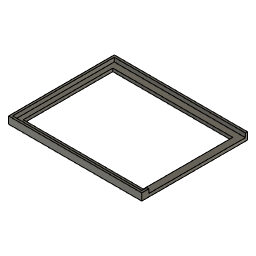
FrontPanel (Autodesk Fusion 360 design; units mm, degrees)
Autodesk Fusion 360 part; units mm, degrees
sketch "Sketch2" plane through (0, 0, 0) normal (0, 0, 1) x (1, 0, 0)
  line L0 (-55.8718, 52.373) -> (71.1282, 52.373)
  line L1 (71.1282, 52.373) -> (71.1282, -47.627)
  line L2 (71.1282, -47.627) -> (-55.8718, -47.627)
  line L3 (-55.8718, -47.627) -> (-55.8718, 52.373)
  line L4 (-51.3718, 46.373) -> (66.6282, 46.373)
  line L5 (66.6282, 46.373) -> (66.6282, -41.627)
  line L6 (66.6282, -41.627) -> (-51.3718, -41.627)
  line L7 (-51.3718, -41.627) -> (-51.3718, 46.373)
  line L8 (-57.8718, 54.373) -> (73.1282, 54.373)
  line L9 (73.1282, 54.373) -> (73.1282, -49.627)
  line L10 (73.1282, -49.627) -> (-57.8718, -49.627)
  line L11 (-57.8718, -49.627) -> (-57.8718, 54.373)
  dimension "d1" = 127
  dimension "d2" = 100
  dimension "d3" = 118
  dimension "d4" = 88
  dimension "d5" = 131
  dimension "d6" = 104
  dimension "d7" = 2
  dimension "d8" = 2
  dimension "d43" = 4.5
  dimension "d44" = 6
  constraint horizontal L0
  constraint vertical L1
  constraint horizontal L2
  constraint vertical L3
  constraint horizontal L4
  constraint vertical L5
  constraint horizontal L6
  constraint vertical L7
  constraint horizontal L8
  constraint vertical L9
  constraint horizontal L10
  constraint vertical L11
  measures "d1" distance of L0.start L0.end
  measures "d2" distance of L0.end L1.end
  measures "d3" distance of L4.start L4.end
  measures "d4" distance of L4.start L6.end
  measures "d5" distance of L8.start L8.end
  measures "d6" distance of L8.start L10.end
  measures "d7" distance of L0 L8
  measures "d8" distance of L3 L11
  measures "d43" distance of L3 L7
  measures "d44" distance of L0 L4
extrude "Extrude7" add sketch "Sketch2" along normal blind 3 contours L0 L1 L2 L3
extrude "Extrude8" add sketch "Sketch2" along normal blind 7 contours L8 L9 L10 L11
sketch "Sketch9" plane through (0, 0, 7) normal (0, 0, 1) x (-1, 0, 0)
  line L0 (-71.1282, 47.627) -> (55.8718, 47.627)
  line L1 (55.8718, 47.627) -> (55.8718, -52.373)
  line L2 (55.8718, -52.373) -> (-71.1282, -52.373)
  line L3 (-71.1282, -52.373) -> (-71.1282, 47.627)
  line L4 (57.8718, 49.627) -> (-73.1282, 49.627)
  line L5 (-73.1282, 49.627) -> (-73.1282, -54.373)
  line L6 (-73.1282, -54.373) -> (57.8718, -54.373)
  line L7 (57.8718, -54.373) -> (57.8718, 49.627)
  line L8 (-71.1282, -52.373) -> (-73.1282, -52.373)
  line L9 (-73.1282, -52.373) -> (-73.1282, 42.627)
  line L10 (-73.1282, 42.627) -> (-71.1282, 42.627)
  line L11 (-71.1282, 42.627) -> (-71.1282, -52.373)
  dimension "d39" = 95
  constraint horizontal L8
  constraint vertical L9
  constraint horizontal L10
  constraint vertical L11
  constraint coincident L5 L9.end
  constraint coincident L2.end L3.start
  measures "d39" distance of L8.end L9.end
extrude "Extrude9" cut sketch "Sketch9" against normal blind 4 contours L3 L5 L8 L9 L10 L11
